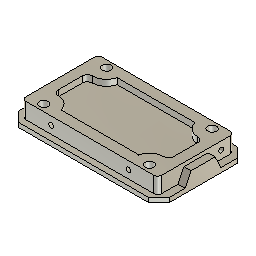
Senso Focuser top cover v3 (Autodesk Fusion 360 design; units mm, degrees)
Autodesk Fusion 360 part; units mm, degrees
sketch "Sketch1" plane through (0, 0, 0) normal (0, 0, 1) x (1, 0, 0)
  line L0 (0, 0) -> (73.72, 0)
  line L1 (73.72, 0) -> (73.72, 43.31)
  line L2 (73.72, 43.31) -> (0, 43.31)
  line L3 (0, 43.31) -> (0, 0)
  dimension "d1" = 73.72
  dimension "d2" = 43.31
  constraint horizontal L0
  constraint vertical L1
  constraint horizontal L2
  constraint vertical L3
  constraint coincident L0.start L3.end
  measures "d1" distance of L0.start L0.end
  measures "d2" distance of L0.start L2.end
extrude "Extrude1" add sketch "Sketch1" along normal blind 10
chamfer "Chamfer1" distance 5 angle 45 4 edges at (73.72, 43.31, 5) (0, 43.31, 5) (73.72, 0, 5) (0, 0, 5)
sketch "Sketch2" plane through (0, 0, 10) normal (0, 0, 1) x (-1, 0, 0)
  line L0 (0, -5) -> (-5, 0)
  line L1 (-5, 0) -> (-68.72, 0)
  line L2 (-68.72, 0) -> (-73.72, -5)
  line L3 (-73.72, -5) -> (-73.72, -38.31)
  line L4 (-73.72, -38.31) -> (-68.72, -43.31)
  line L5 (-68.72, -43.31) -> (-5, -43.31)
  line L6 (-5, -43.31) -> (0, -38.31)
  line L7 (0, -38.31) -> (0, -5)
  line L8 (0, -21.655) -> (-73.72, -21.655) construction
  line L9 (-36.86, -43.31) -> (-36.86, 0) construction
  line L10 (-5.495, -40.41) -> (-68.225, -40.41)
  line L11 (-70.225, -38.41) -> (-70.225, -4.9)
  line L12 (-68.225, -2.9) -> (-5.495, -2.9)
  line L13 (-3.495, -4.9) -> (-3.495, -38.41)
  line L14 (-3.495, -40.41) -> (-70.225, -2.9) construction
  line L15 (-70.225, -40.41) -> (-3.495, -2.9) construction
  arc A0 (-5.495, -40.41) -> (-3.495, -38.41) centre (-5.495, -38.41) ccw
  arc A1 (-70.225, -38.41) -> (-68.225, -40.41) centre (-68.225, -38.41) ccw
  arc A2 (-68.225, -2.9) -> (-70.225, -4.9) centre (-68.225, -4.9) ccw
  arc A3 (-3.495, -4.9) -> (-5.495, -2.9) centre (-5.495, -4.9) ccw
  point P0 (-36.86, -21.655)
  dimension "d6" = 37.51
  dimension "d7" = 66.73
  dimension "d8" = 2
  constraint midpoint L7 L8.start
  constraint midpoint L3 L8.end
  constraint midpoint L5 L9.start
  constraint midpoint L1 L9.end
  constraint horizontal L10
  constraint perpendicular L10 L11
  constraint parallel L10 L12
  constraint parallel L11 L13
  constraint coincident L14 P0
  constraint coincident L15 P0
  constraint midpoint L9 P0
  constraint coincident L14.start L13
  constraint coincident L14.start L10
  constraint tangent L13 A0
  constraint tangent L10 A0
  constraint coincident L15.start L10
  constraint coincident L15.start L11
  constraint tangent L10 A1
  constraint tangent L11 A1
  constraint equal A0 A1
  constraint coincident L14.end L11
  constraint coincident L14.end L12
  constraint tangent L11 A2
  constraint tangent L12 A2
  constraint equal A0 A2
  constraint coincident L15.end L12
  constraint coincident L15.end L13
  constraint tangent L12 A3
  constraint tangent L13 A3
  constraint equal A0 A3
  measures "d6" distance of L15.start L14.end
  measures "d7" distance of L14.end L15.end
  measures "d8" radius of A0
extrude "Extrude2" cut sketch "Sketch2" against normal blind 7.9
sketch "Sketch3" plane through (0, 0, 2.1) normal (0, 0, 1) x (-1, 0, 0)
  arc A0 (-5.495, -40.41) -> (-3.495, -38.41) centre (-5.495, -38.41) ccw
  line L0 (-5.495, -40.41) -> (-68.225, -40.41)
  arc A1 (-70.225, -38.41) -> (-68.225, -40.41) centre (-68.225, -38.41) ccw
  line L1 (-70.225, -38.41) -> (-70.225, -4.9)
  arc A2 (-68.225, -2.9) -> (-70.225, -4.9) centre (-68.225, -4.9) ccw
  line L2 (-68.225, -2.9) -> (-5.495, -2.9)
  arc A3 (-3.495, -4.9) -> (-5.495, -2.9) centre (-5.495, -4.9) ccw
  line L3 (-3.495, -4.9) -> (-3.495, -38.41)
  line L4 (0, -38.31) -> (0, -5)
  line L5 (0, -5) -> (-5, 0)
  line L6 (-5, 0) -> (-68.72, 0)
  line L7 (-68.72, 0) -> (-73.72, -5)
  line L8 (-73.72, -5) -> (-73.72, -38.31)
  line L9 (-73.72, -38.31) -> (-68.72, -43.31)
  line L10 (-68.72, -43.31) -> (-5, -43.31)
  line L11 (-5, -43.31) -> (0, -38.31)
  line L12 (-73.72, -21.655) -> (0, -21.655) construction
  line L13 (-73.72, -12.885) -> (-70.225, -12.885)
  line L14 (-73.72, -30.425) -> (-70.225, -30.425)
  dimension "d11" = 8.77
  dimension "d12" = 8.77
  constraint midpoint L8 L12.start
  constraint midpoint L4 L12.end
  constraint coincident L8 L13.start
  constraint coincident L1 L13.end
  constraint perpendicular L1 L13
  constraint coincident L8 L14.start
  constraint coincident L1 L14.end
  constraint perpendicular L1 L14
  measures "d11" distance of L12 L13
  measures "d12" distance of L12 L14
extrude "Extrude3" add sketch "Sketch3" along normal blind 5.9 contours L1 L8 L13 L14
chamfer "Chamfer2" distance 2.95 distance2 5.9 2 edges at (71.9725, 12.885, 8) (71.9725, 30.425, 8) measured on face at (71.39, 18.7317, 8) measured on face at (71.39, 18.7317, 8)
sketch "Sketch4" plane through (0, 0, 10) normal (0, 0, 1) x (-1, 0, 0)
  line L0 (-68.225, -40.41) -> (-5.495, -40.41)
  arc A0 (-5.495, -40.41) -> (-3.495, -38.41) centre (-5.495, -38.41) ccw
  line L1 (-3.495, -38.41) -> (-3.495, -4.9)
  arc A1 (-3.495, -4.9) -> (-5.495, -2.9) centre (-5.495, -4.9) ccw
  line L2 (-5.495, -2.9) -> (-68.225, -2.9)
  arc A2 (-68.225, -2.9) -> (-70.225, -4.9) centre (-68.225, -4.9) ccw
  line L3 (-70.225, -4.9) -> (-70.225, -38.41)
  arc A3 (-70.225, -38.41) -> (-68.225, -40.41) centre (-68.225, -38.41) ccw
  line L4 (-3.495, -21.655) -> (-70.225, -21.655) construction
  line L5 (-36.86, -40.41) -> (-36.86, -2.9) construction
  line L6 (-10.96, -37.055) -> (-62.76, -37.055) construction
  line L7 (-62.76, -37.055) -> (-62.76, -6.255) construction
  line L8 (-62.76, -6.255) -> (-10.96, -6.255) construction
  line L9 (-10.96, -6.255) -> (-10.96, -37.055) construction
  line L10 (-10.96, -37.055) -> (-62.76, -6.255) construction
  line L11 (-62.76, -37.055) -> (-10.96, -6.255) construction
  circle A4 centre (-10.96, -37.055) radius 2.15
  circle A5 centre (-62.76, -37.055) radius 2.15
  circle A6 centre (-62.76, -6.255) radius 2.15
  circle A7 centre (-10.96, -6.255) radius 2.15
  circle A8 centre (-10.96, -37.055) radius 3.355
  circle A9 centre (-62.76, -37.055) radius 3.355
  circle A10 centre (-62.76, -6.255) radius 3.355
  circle A11 centre (-10.96, -6.255) radius 3.355
  circle A12 centre (-10.96, -37.055) radius 4
  circle A13 centre (-62.76, -37.055) radius 4
  circle A14 centre (-62.76, -6.255) radius 4
  circle A15 centre (-10.96, -6.255) radius 4
  point P0 (-36.86, -21.655)
  dimension "d17" = 30.8
  dimension "d18" = 51.8
  dimension "d19" = 4.3
  dimension "d20" = 4.3
  dimension "d21" = 4.3
  dimension "d22" = 4.3
  dimension "d27" = 8
  dimension "d28" = 8
  dimension "d29" = 8
  dimension "d30" = 8
  constraint midpoint L1 L4.start
  constraint midpoint L3 L4.end
  constraint midpoint L0 L5.start
  constraint midpoint L2 L5.end
  constraint horizontal L6
  constraint perpendicular L6 L7
  constraint parallel L6 L8
  constraint parallel L7 L9
  constraint coincident L10 P0
  constraint coincident L11 P0
  constraint midpoint L5 P0
  constraint coincident L6.start L9.end
  constraint coincident L6.end L7.start
  constraint coincident L7.end L8.start
  constraint coincident L8.end L9.start
  constraint concentric A4 A8
  constraint tangent L0 A8
  constraint concentric A5 A9
  constraint tangent L0 A9
  constraint concentric A6 A10
  constraint tangent L2 A10
  constraint concentric A7 A11
  constraint tangent L2 A11
  constraint concentric A4 A12
  constraint concentric A9 A13
  constraint concentric A6 A14
  constraint concentric A11 A15
  measures "d17" distance of L6.start L8.end
  measures "d18" distance of L7.end L8.end
  measures "d19" diameter of A4
  measures "d20" diameter of A7
  measures "d21" diameter of A5
  measures "d22" diameter of A6
  measures "d27" diameter of A12
  measures "d28" diameter of A13
  measures "d29" diameter of A14
  measures "d30" diameter of A15
extrude "Extrude4" cut sketch "Sketch4" against normal blind 1 contours L0 A0 L1 A1 L2 A2 L3 A3 A12 A13 A14 A15 | L0 A13 | L0 A12 | L2 A14 | L2 A15 picked at (-64.9901, -40.1025) picked at (-13.1901, -40.1025) picked at (-64.9901, -3.2075) picked at (-13.1901, -3.2075)
extrude "Extrude5" cut sketch "Sketch4" against normal blind 6 contours A4 | A5 | A6 | A7
sketch "Sketch5" plane through (0, 2.9, 0) normal (0, -1, 0) x (1, 0, 0)
  line L0 (68.225, 9) -> (62.76, 9)
  line L1 (5.495, 9) -> (5.495, 2.1)
  line L2 (5.495, 2.1) -> (68.225, 2.1)
  line L3 (68.225, 2.1) -> (68.225, 9)
  circle A0 centre (55.86, 6.1) radius 1.15
  circle A1 centre (17.86, 6.1) radius 1.15
  line L4 (36.86, 8) -> (36.86, 2.1) construction
  line L5 (68.72, 0) -> (5, 0)
  line L6 (62.76, 9) -> (10.96, 9)
  line L7 (10.96, 9) -> (5.495, 9)
  dimension "d31" = 2.3
  dimension "d32" = 2.3
  dimension "d33" = 19
  dimension "d34" = 19
  dimension "d42" = 6.1
  constraint midpoint L2 L4.end
  measures "d31" diameter of A0
  measures "d32" diameter of A1
  measures "d33" distance of A0.centre L4
  measures "d34" distance of A1.centre L4
  measures "d42" distance of A1.centre L5
sketch "Sketch6" plane through (70.225, 0, 0) normal (1, 0, 0) x (0, 1, 0)
  line L0 (38.41, 9) -> (4.9, 9)
  line L1 (27.475, 8) -> (30.425, 2.1)
  line L2 (4.9, 2.1) -> (12.885, 2.1)
  line L3 (38.41, 2.1) -> (38.41, 9)
  circle A0 centre (34.01, 6.1) radius 1.15
  line L4 (43.31, 0) -> (43.31, 2.1)
  line L5 (5, 0) -> (38.31, 0)
  line L6 (4.9, 9) -> (4.9, 2.1)
  line L7 (12.885, 2.1) -> (15.835, 8)
  line L8 (15.835, 8) -> (27.475, 8)
  line L9 (30.425, 2.1) -> (38.41, 2.1)
  dimension "d35" = 2.3
  dimension "d36" = 9.3
  dimension "d37" = 6.1
  measures "d35" diameter of A0
  measures "d36" distance of A0.centre L4
  measures "d37" distance of A0.centre L5
sketch "Sketch7" plane through (3.495, 0, 0) normal (-1, 0, 0) x (0, -1, 0)
  line L0 (-4.9, 9) -> (-38.41, 9)
  line L1 (-38.41, 9) -> (-38.41, 2.1)
  line L2 (-38.41, 2.1) -> (-4.9, 2.1)
  line L3 (-4.9, 2.1) -> (-4.9, 9)
  circle A0 centre (-34.01, 6.1) radius 1.15
extrude "Extrude6" cut sketch "Sketch7" against normal blind 3.5 contours A0
extrude "Extrude7" cut sketch "Sketch6" against normal blind 3.5 contours A0
extrude "Extrude8" cut sketch "Sketch5" against normal blind 5 contours A0 | A1
extrude "Extrude9" add sketch "Sketch4" against normal blind 1 contours L0 A12 picked at (-13.1901, -40.1025)
extrude "Extrude10" add sketch "Sketch4" against normal blind 1 contours L0 A13 picked at (-64.9901, -40.1025)
extrude "Extrude11" add sketch "Sketch4" against normal blind 1 contours L2 A14 | L2 A15 picked at (-64.9901, -3.2075) picked at (-13.1901, -3.2075)
sketch "Sketch8" plane through (0, 0, 9) normal (0, 0, 1) x (-1, 0, 0)
  arc A0 (-13.1381, -2.9) -> (-8.7819, -2.9) centre (-10.96, -6.255) ccw
  line L0 (-13.1381, -2.9) -> (-60.5819, -2.9)
  arc A1 (-64.9381, -2.9) -> (-60.5819, -2.9) centre (-62.76, -6.255) ccw
  line L1 (-64.9381, -2.9) -> (-68.225, -2.9)
  arc A2 (-68.225, -2.9) -> (-70.225, -4.9) centre (-68.225, -4.9) ccw
  line L2 (-70.225, -4.9) -> (-70.225, -38.41)
  arc A3 (-70.225, -38.41) -> (-68.225, -40.41) centre (-68.225, -38.41) ccw
  line L3 (-68.225, -40.41) -> (-64.9381, -40.41)
  arc A4 (-60.5819, -40.41) -> (-64.9381, -40.41) centre (-62.76, -37.055) ccw
  line L4 (-60.5819, -40.41) -> (-13.1381, -40.41)
  arc A5 (-8.7819, -40.41) -> (-13.1381, -40.41) centre (-10.96, -37.055) ccw
  line L5 (-8.7819, -40.41) -> (-5.495, -40.41)
  arc A6 (-5.495, -40.41) -> (-3.495, -38.41) centre (-5.495, -38.41) ccw
  line L6 (-3.495, -38.41) -> (-3.495, -4.9)
  arc A7 (-3.495, -4.9) -> (-5.495, -2.9) centre (-5.495, -4.9) ccw
  line L7 (-5.495, -2.9) -> (-8.7819, -2.9)
  arc A8 (-8.495, -28.3991) -> (-19.8084, -35.41) centre (-10.96, -37.055) ccw
  line L8 (-53.9116, -35.41) -> (-19.8084, -35.41)
  arc A9 (-53.9116, -35.41) -> (-65.225, -28.3991) centre (-62.76, -37.055) ccw
  line L9 (-65.225, -14.9109) -> (-65.225, -28.3991)
  arc A10 (-65.225, -14.9109) -> (-53.9116, -7.9) centre (-62.76, -6.255) ccw
  line L10 (-19.8084, -7.9) -> (-53.9116, -7.9)
  arc A11 (-19.8084, -7.9) -> (-8.495, -14.9109) centre (-10.96, -6.255) ccw
  line L11 (-8.495, -28.3991) -> (-8.495, -14.9109)
  dimension "d51" = -5
extrude "Extrude12" cut sketch "Sketch8" against normal blind 2 contours A8 L8 A9 L9 A10 L10 A11 L11
extrude "Extrude13" add 2 faces at (72.555, 30.425, 2.1004) (72.555, 28.4587, 6.0337) along direction (0, 0.894427, 0.447214) blind 0.05
extrude "Extrude14" add 2 faces at (71.39, 12.885, 2.1004) (72.555, 14.8513, 6.0337) along direction (0, -0.894427, 0.447214) blind 0.05
ref_plane "WorkPlane1" through (71.9725, 21.655, 9) normal (0, 0, 1) x (1, 0, 0)
sketch "Sketch9" plane through (0, 0, 9) normal (0, 0, 1) x (1, 0, 0)
  line L0 (73.72, 27.5197) -> (73.72, 30.4697)
  line L1 (73.72, 30.4697) -> (70.225, 30.4697)
  line L2 (70.225, 30.4697) -> (70.225, 27.5197)
  line L3 (70.225, 27.5197) -> (73.72, 27.5197)
  line L4 (73.72, 12.8403) -> (73.72, 15.7903)
  line L5 (73.72, 15.7903) -> (70.225, 15.7903)
  line L6 (70.225, 15.7903) -> (70.225, 12.8403)
  line L7 (70.225, 12.8403) -> (73.72, 12.8403)
  line L8 (73.72, 27.475) -> (70.225, 27.475)
  line L9 (70.225, 27.475) -> (70.225, 15.835)
  line L10 (70.225, 15.835) -> (73.72, 15.835)
  line L11 (73.72, 15.835) -> (73.72, 27.475)
  line L12 (70.225, 27.475) -> (73.72, 27.475)
  line L13 (73.72, 27.475) -> (73.72, 27.5197)
  line L14 (73.72, 27.5197) -> (70.225, 27.5197)
  line L15 (70.225, 27.5197) -> (70.225, 27.475)
  line L16 (73.72, 15.835) -> (70.225, 15.835)
  line L17 (70.225, 15.835) -> (70.225, 15.7903)
  line L18 (70.225, 15.7903) -> (73.72, 15.7903)
  line L19 (73.72, 15.7903) -> (73.72, 15.835)
extrude "Extrude15" cut sketch "Sketch9" against normal blind 1
fillet "Fillet1" radius 0.5 2 edges at (71.9725, 15.7791, 8) (71.9725, 27.5309, 8)
extrude "Extrude16" add 1 faces at (2.33, 16.1033, 2.1) along direction (0, 0, 1) blind 0.1
extrude "Extrude17" cut 1 faces at (66.725, 33.868, 6.4823) along direction (-1, 0, 0) blind 0.5
extrude "Extrude18" cut 1 faces at (6.995, 34.152, 6.4823) along direction (1, 0, 0) blind 1
extrude "Extrude19" cut 1 faces at (68.5583, 19.407, 9) along direction (0, 0, -1) blind 1
extrude "Extrude20" add 1 faces at (5.1617, 19.407, 8) along direction (0, 0, 1) blind 2
move_face "OffsetFaces1" offset -2 4 faces at (19.7229, 35.0028, 9) (64.8223, 28.2945, 9) (59.8981, 14.7879, 9) (18.8259, 10.6285, 8)
fillet "Fillet2" radius 2.5 4 edges at (65.225, 30.5034, 8.5) (65.225, 12.8066, 8.5) (8.495, 30.5034, 8.5) (8.495, 12.8066, 8.5)
extrude "Extrude21" cut sketch "Sketch9" along normal blind 2.5 and the other way blind 1.25
extrude "Extrude22" cut sketch "Sketch9" against normal blind 6.8
sketch "Sketch10" plane through (0, 0, 2.2) normal (0, 0, 1) x (-1, 0, 0)
  line L0 (-70.225, -38.41) -> (-70.225, -4.9)
  arc A0 (-68.225, -2.9) -> (-70.225, -4.9) centre (-68.225, -4.9) ccw
  line L1 (-68.225, -2.9) -> (-5.495, -2.9)
  arc A1 (-3.495, -4.9) -> (-5.495, -2.9) centre (-5.495, -4.9) ccw
  line L2 (-3.495, -4.9) -> (-3.495, -38.41)
  arc A2 (-5.495, -40.41) -> (-3.495, -38.41) centre (-5.495, -38.41) ccw
  line L3 (-5.495, -40.41) -> (-68.225, -40.41)
  arc A3 (-70.225, -38.41) -> (-68.225, -40.41) centre (-68.225, -38.41) ccw
  line L4 (-73.72, -5) -> (-73.72, -38.31)
  line L5 (-73.72, -38.31) -> (-68.72, -43.31)
  line L6 (-68.72, -43.31) -> (-5, -43.31)
  line L7 (-5, -43.31) -> (0, -38.31)
  line L8 (0, -38.31) -> (0, -5)
  line L9 (0, -5) -> (-5, 0)
  line L10 (-5, 0) -> (-68.72, 0)
  line L11 (-68.72, 0) -> (-73.72, -5)
  line L12 (-70.225, -21.655) -> (-73.72, -21.655) construction
  line L13 (-73.72, -30.455) -> (-70.225, -30.455)
  line L14 (-70.225, -12.855) -> (-73.72, -12.855)
  dimension "d84" = 8.8
  dimension "d85" = 8.8
  constraint midpoint L0 L12.start
  constraint midpoint L4 L12.end
  constraint coincident L4 L13.start
  constraint coincident L0 L13.end
  constraint perpendicular L0 L13
  constraint coincident L0 L14.start
  constraint coincident L4 L14.end
  constraint perpendicular L4 L14
  measures "d84" distance of L12 L13
  measures "d85" distance of L12 L14
extrude "Extrude23" add sketch "Sketch10" along normal blind 6 contours L0 L4 L13 L14
chamfer "Chamfer3" distance 2.9 distance2 6 2 edges at (71.9725, 12.855, 8.2) (71.9725, 30.455, 8.2) measured on face at (71.39, 24.5883, 8.2) measured on face at (71.39, 24.5883, 8.2)
equation "d11 = ( 17.54 / 2 ) * 1 mm"
equation "d12 = d11"
equation "d19 = pcb_mtg"
equation "d20 = pcb_mtg"
equation "d21 = pcb_mtg"
equation "d22 = pcb_mtg"
equation "d31 = covr_scrw"
equation "d32 = covr_scrw"
equation "d35 = covr_scrw"
equation "covr_scrw = 2.3 mm" comment "side holes for self taping cover screws"
equation "pcb_mtg = 4.3 mm"
equation "d84 = ( 17.6 / 2 ) * 1 mm"
equation "d85 = d84"
equation "d89 = Distance 2"
